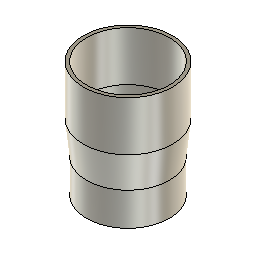
Absaugadapter parametrisch v1 (Autodesk Fusion 360 design; units mm, degrees)
Autodesk Fusion 360 part; units mm, degrees
note: some values were not read from the file. Set by a fixed rule: which face or edge a step refers to.
sketch "Skizze1" plane through (0, 0, 0) normal (0, 0, 1) x (1, 0, 0)
  circle A0 centre (0, 0) radius 25
  circle A1 centre (0, 0) radius 23
  dimension "d1" = 50
  dimension "d2" = 46
  constraint coincident A0.centre A1.centre
  measures "d1" diameter of A0
  measures "d2" diameter of A1
extrude "Extrusion1" add sketch "Skizze1" along normal blind 20 contours A0 | A1
ref_plane "Arbeitsebene1" through (0, 0, 40) normal (0, 0, 1) x (1, 0, 0)
sketch "Skizze2" plane through (0, 0, 40) normal (0, 0, 1) x (1, 0, 0)
  circle A0 centre (0, 0) radius 27
  dimension "d8" = 54
  constraint coincident A0.centre origin
  measures "d8" diameter of A0
loft "Erhebung1" add profiles "Skizze2" section 1 face at (-4.9866, 5.1277, 20) section 2
extrude "Extrusion2" add 1 faces at (4.1002, 2.99, 40) along direction (0, 0, 1) blind 30
shell "Schale1" thickness 2 removed faces 1 at (-4.9866, 5.1277, 0)
delete_face "Fläche löschen1" 1 faces at (-5.5413, -1.9035, 68)
ref_plane "Arbeitsebene2" through (0, 0, 2) normal (0, 0, 1) x (1, 0, 0)
sketch "Skizze4" plane through (0, 0, 2) normal (0, 0, 1) x (1, 0, 0)
  circle A0 centre (0, 0) radius 25
  circle A1 centre (0, 0) radius 18
  dimension "d14" = 50
  dimension "d15" = 36
  constraint coincident A0.centre A1.centre
  measures "d14" diameter of A0
  measures "d15" diameter of A1
extrude "Extrusion3" add sketch "Skizze4" along normal blind 2
equation "Height_mm = 30 mm"
equation "inner_Diameter_mm = 50 mm"
equation "d8 = inner_Diameter_mm + 4 mm"
equation "d10 = Height_mm"
